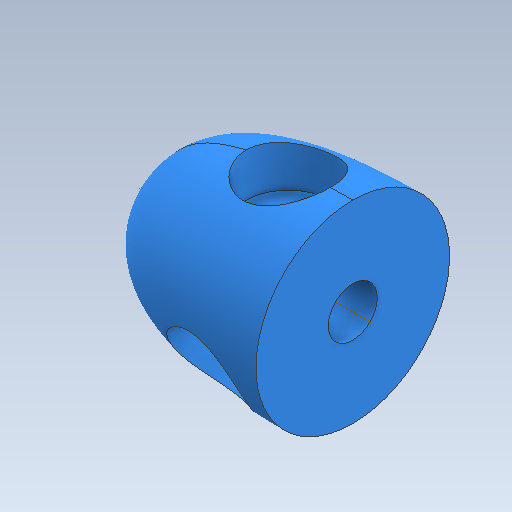
# Autodesk Inventor part: Rotor
Saved by Autodesk Inventor 2021 (Build 250183000, 183)
## iProperties
Created: 2022-01-11
Part Number: Rotor
Material: Iron, Malleable
Document SubType Name: Modeling
Designer: stefi
Density: 7.15 g/cm^3
Appearance: Semi-Polished
Author: stefi
Autodesk Inventor part; units mm, degrees
ref_plane "YZ Plane" through (0, 0, 0) normal (1, 0, 0) x (0, 1, 0)
ref_plane "XY Plane" through (0, 0, 0) normal (0, 0, 1) x (1, 0, 0)
sketch "Sketch1" plane through (0, 0, 0) normal (0, 0, 1) x (1, 0, 0)
  line L0 (0, 0) -> (-38.1, 0)
  line L1 (0, 0) -> (0, 19.05)
  line L2 (0, 19.05) -> (-26.0241, 19.05) construction
  spline S0 degree 3 poles (0, 19.05) (-26.0241, 19.05) (-38.1, 12.9916) (-38.1, 0) knots 1 1 1 1 2 2 2 2
  line L3 (-38.1, 12.9916) -> (-38.1, 0) construction
  line L4 (-26.0241, 19.05) -> (-38.1, 12.9916) construction
  dimension "d0" = 38.1
  dimension "d1" = 19.05
  constraints: 4 end point, 2 horizontal, 2 vertical, 3 other
  measures "d0" distance of L0.start L0.end
  measures "d1" distance of L0.start L1.end
revolve "Revolution1" add sketch "Sketch1" angle 360 about axis through (0, 0, 0) along (-1, 0, 0)
ref_plane "Work Plane1" through (0, 20, 0) normal (0, 1, 0) x (-1, 0, 0)
sketch "Sketch2" plane through (0, 20, 0) normal (0, 1, 0) x (-1, 0, 0)
  circle A0 centre (12.7, 0) radius 8.26
  line L0 (0, 0) -> (12.7, 0)
  dimension "d4" = 12.7
  dimension "d5" = 16.52
  constraints: 2 end point, 1 centre point, 1 horizontal
  measures "d4" distance of L0.start L0.end
  measures "d5" diameter of A0
extrude "Extrusion1" cut sketch "Sketch2" against normal blind 11.43
pattern_circular "Circular Pattern1" count 3 over 360 about axis through (-10, 0, 0) along (1, 0, 0) of "Extrusion1"
sketch "Sketch3" plane through (0, 0, 0) normal (1, 0, 0) x (0, 0, -1)
  circle A0 centre (0, 0) radius 4.826
  dimension "d11" = 9.652
  constraints: 1 centre point, 1 coincident
  measures "d11" diameter of A0
extrude "Extrusion2" cut sketch "Sketch3" against normal blind 12.7
body "Solid1"
